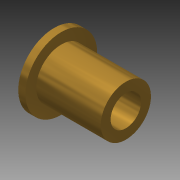
# Autodesk Inventor part: Output Shaft Insert
Saved by Autodesk Inventor 2013 (Build 170138000, 138)
## iProperties
Created: 2013-06-06
Part Number: Output Shaft Insert
Material: Generic
Document SubType Name: Modeling
Designer: mvarma
Density: 1 g/cm^3
Author: mvarma
Autodesk Inventor part; units mm, degrees
ref_plane "YZ Plane" through (0, 0, 0) normal (1, 0, 0) x (0, 1, 0)
ref_plane "XZ Plane" through (0, 0, 0) normal (0, 1, 0) x (-1, 0, 0)
ref_plane "XY Plane" through (0, 0, 0) normal (0, 0, 1) x (1, 0, 0)
sketch "Sketch1" plane through (0, 0, 0) normal (0, 0, 1) x (1, 0, 0)
  line L0 (0, 0) -> (0, 12.7) construction
  line L1 (0, 5.5563) -> (5.5562, 5.5563)
  line L2 (0, 7.9375) -> (26.1937, 7.9375) construction
  line L3 (26.1937, 7.9375) -> (26.1937, 5.5563) construction
  line L4 (26.1937, 5.5563) -> (26.1937, 0) construction
  line L5 (26.1937, 0) -> (0, 0) construction
  line L6 (26.1938, 6.35) -> (34.3852, 6.35) construction
  line L7 (26.1937, 0) -> (34.3852, 0) construction
  line L8 (34.3852, 0) -> (34.3852, 6.35) construction
  line L9 (16.6687, 7.9375) -> (16.6687, 0) construction
  circle A0 centre (16.6687, 7.5565) radius 2.3813 construction
  circle A1 centre (16.6687, 5.4928) radius 2.3813 construction
  circle A2 centre (10.3187, 7.5565) radius 2.3813 construction
  circle A3 centre (10.3187, 5.4928) radius 2.3813 construction
  line L10 (10.3187, 7.9375) -> (10.3187, 0) construction
  line L11 (0, 5.1753) -> (26.1938, 5.1753) construction
  line L12 (8.7312, 5.1753) -> (8.7312, 0) construction
  line L13 (5.5562, 5.1753) -> (5.5562, 3.3734)
  line L14 (18.2562, 5.1753) -> (18.2562, 0) construction
  line L15 (21.4312, 5.1753) -> (21.4312, 0) construction
  line L16 (0, 3.1115) -> (26.1937, 3.1115) construction
  line L17 (5.5562, 3.1115) -> (8.7312, 5.1753) construction
  line L18 (18.2562, 5.1753) -> (21.4312, 3.1115) construction
  line L19 (11.9062, 5.1753) -> (11.9062, 0) construction
  line L20 (15.0812, 5.1753) -> (15.0812, 0) construction
  line L21 (11.9062, 5.1753) -> (15.0812, 3.1115) construction
  line L22 (21.4312, 3.3734) -> (34.3852, 3.3734) construction
  line L23 (24.6062, 3.3734) -> (24.6062, 0) construction
  line L24 (21.4312, 3.3734) -> (20.1197, 5.5563) construction
  line L25 (26.1937, 3.1115) -> (30.9563, 3.1115) construction
  line L26 (30.9563, 3.1115) -> (30.9563, 0) construction
  line L27 (31.75, 3.3734) -> (31.75, 0) construction
  line L28 (31.75, 0) -> (29.723, 3.3734) construction
  line L29 (0, 7.9375) -> (-8.7312, 7.9375) construction
  line L30 (0, 3.3734) -> (5.5562, 3.3734)
  line L31 (5.5562, 5.1753) -> (5.5562, 5.5563)
  line L32 (5.5562, 5.5563) -> (26.1937, 5.5563) construction
  line L33 (0, 5.5563) -> (-8.7312, 5.5562)
  line L34 (-10.3187, 7.9375) -> (-10.3187, 3.3734)
  line L35 (-10.3187, 3.3734) -> (0, 3.3734)
  line L36 (-8.7312, 7.9375) -> (-8.7312, 5.5562)
  line L37 (-8.7312, 7.9375) -> (-10.3187, 7.9375)
  line L38 (5.5562, 3.3734) -> (5.5562, 0) construction
  dimension "d0" = 12.7
  dimension "d1" = 5.5563
  dimension "d2" = 7.9375
  dimension "d3" = 26.1938
  dimension "d4" = 8.1915
  dimension "d5" = 6.35
  dimension "d6" = 9.525
  dimension "d7" = 6.35
  dimension "d8" = 0.381
  dimension "d9" = 0.381
  dimension "d10" = 0.0635
  dimension "d11" = 0.0635
  dimension "d12" = 1.5875
  dimension "d13" = 4.7625
  dimension "d14" = 1.5875
  dimension "d15" = 4.7625
  dimension "d16" = 3.1115
  dimension "d17" = 1.5875
  dimension "d18" = 4.7625
  dimension "d19" = 3.3734
  dimension "d20" = 3.175
  dimension "d21" = 31
  dimension "d22" = 9.525
  dimension "d23" = 9.525
  dimension "d24" = 0.7937
  dimension "d25" = 31
  dimension "d27" = 3.3734
  dimension "d33" = 4.7625
  dimension "d34" = 8.7312
  dimension "d35" = 1.5875
  constraints: 77 end point, 36 point on line, 17 perpendicular, 12 vertical, 4 centre point, 4 coincident, 3 equal radius, 3 parallel, 2 horizontal, 2 tangent, 1 collinear, 12 other
  measures "d0" distance of L0.start L0.end
  measures "d1" distance from line of L1 L0.start
  measures "d2" distance from line of L0.start L2
  measures "d3" distance of L2.start L2.end
  measures "d4" distance of L6.start L6.end
  measures "d5" distance of L7.end L6.end
  measures "d6" distance between parallel lines of L3 L9
  measures "d7" distance between parallel lines of L9 L10
  measures "d8" distance from line of L2 A2.centre
  measures "d9" distance from line of L2 A0.centre
  measures "d10" distance from line of L1 A1.centre
  measures "d11" distance from line of L1 A3.centre
  measures "d12" distance between parallel lines of L12 L10
  measures "d13" distance between parallel lines of L13 L10
  measures "d14" distance between parallel lines of L9 L14
  measures "d15" distance between parallel lines of L15 L9
  measures "d16" distance of the line from the sketch origin of L16
  measures "d17" distance between parallel lines of L10 L19
  measures "d18" distance between parallel lines of L10 L20
  measures "d19" distance between parallel lines of L7 L22
  measures "d20" distance between parallel lines of L15 L23
  measures "d21" angle of L15 L24
  measures "d22" distance from line of L23 L21.end
  measures "d23" distance from line of L26 L18.end
  measures "d24" distance between parallel lines of L27 L26
  measures "d25" angle of L27 L28
  measures "d27" distance of the line from the sketch origin of L30
  measures "d33" diameter of A2
  measures "d34" distance of L2.start L29.end
  measures "d35" distance of L29.end L34.start
revolve "Revolution1" add sketch "Sketch1" angle 360 about axis through (26.1937, 0, 0) along (-1, 0, 0)
equation "\"d1\" = d28"
equation "\"d2\" = d29"
equation "\"d8\" = d30"
equation "\"d9\" = d8"
equation "\"d10\" = d31"
equation "\"d11\" = d10"
equation "\"d16\" = d32"
equation "\"d17\" = d12"
equation "\"d18\" = d13"
equation "\"d23\" = d22"
equation "\"d25\" = d21"
equation "\"d27\" = d19"
equation "\"d28\" = 5.55625"
equation "\"d29\" = 7.9375"
equation "\"d30\" = 0.381"
equation "\"d31\" = 0.0635"
equation "\"d32\" = 3.1115"
body "Solid1"
